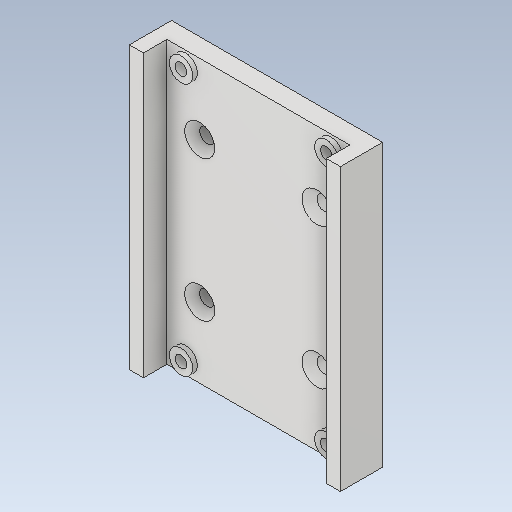
# Autodesk Inventor part: 회로프레임
Saved by Autodesk Inventor 2020.5 (Build 245400000, 400)
## iProperties
Created: 2021-07-21
Part Number: 회로프레임
Material: LCP 플라스틱
Document SubType Name: Modeling
Designer: user
Density: 1.626 g/cm^3
Appearance: 매끄러움 - 흰색
Mass: 20.1348 g
Surface Area: 77.5279 cm^2
Volume: 12.3831 cm^3
Author: user
Autodesk Inventor part; units mm, degrees
ref_plane "YZ Plane" through (0, 0, 0) normal (1, 0, 0) x (0, 1, 0)
ref_plane "XZ Plane" through (0, 0, 0) normal (0, 1, 0) x (-1, 0, 0)
ref_plane "XY Plane" through (0, 0, 0) normal (0, 0, 1) x (1, 0, 0)
sketch "스케치1" plane through (0, 0, 0) normal (0, 0, 1) x (1, 0, 0)
  line L0 (-22.5, 30) -> (22.5, 30)
  line L1 (22.5, 30) -> (22.5, -30)
  line L2 (22.5, -30) -> (-22.5, -30)
  line L3 (-22.5, -30) -> (-22.5, 30)
  point P0 (0, 0)
  dimension "d0" = 45
  dimension "d1" = 60
  dimension "d2" = 30
  dimension "d3" = 22.5
  constraints: 8 end point, 2 parallel, 1 horizontal, 1 perpendicular
  measures "d0" distance of L1.end L2.end
  measures "d1" distance of L0.end L1.end
  measures "d2" distance from line of L0 point (0, 0)
  measures "d3" distance from line of L3 point (0, 0)
extrude "돌출1" add sketch "스케치1" along normal blind 4
sketch "스케치2" plane through (0, 0, 4) normal (0, 0, 1) x (1, 0, 0)
  line L0 (-15.5, 27) -> (15.5, 27)
  line L1 (15.5, 27) -> (15.5, -27)
  line L2 (15.5, -27) -> (-15.5, -27)
  line L3 (-15.5, -27) -> (-15.5, 27)
  circle A0 centre (-15.5, 27) radius 1.25
  circle A1 centre (15.5, 27) radius 1.25
  circle A2 centre (-15.5, -27) radius 1.25
  circle A3 centre (15.5, -27) radius 1.25
  point P0 (0, 0)
  dimension "d6" = 31
  dimension "d7" = 54
  dimension "d8" = 15.5
  dimension "d9" = 27
  dimension "d10" = 2.5
  dimension "d11" = 2.5
  dimension "d12" = 2.5
  dimension "d13" = 2.5
  constraints: 8 end point, 4 centre point, 4 coincident, 2 parallel, 1 horizontal, 1 perpendicular
  measures "d6" distance between parallel lines of L1 L3
  measures "d7" distance between parallel lines of L2 L0
  measures "d8" distance from line of L3 point (0, 0)
  measures "d9" distance from line of point (0, 0) L0
  measures "d10" diameter of A0
  measures "d11" diameter of A1
  measures "d12" diameter of A2
  measures "d13" diameter of A3
extrude "돌출2" cut sketch "스케치2" against normal up to surface (4 mm away) contours L3 A0 L0 | L0 A0 L3 | A1 L1 L0 | L0 L1 A1 | A2 L2 L3 | L3 L2 A2 | A3 L2 L1 | L1 L2 A3
sketch "스케치3" plane through (0, 0, 4) normal (0, 0, 1) x (1, 0, 0)
  line L0 (-22.5, 30) -> (-22.5, -30) projected
  line L1 (-22.5, -30) -> (22.5, -30) projected
  line L2 (-22.5, 30) -> (-19.5, 30)
  line L3 (-19.5, 30) -> (-19.5, -30)
  line L4 (-19.5, -30) -> (-22.5, -30)
  line L5 (-22.5, -30) -> (-22.5, 30)
  line L6 (22.5, 30) -> (-22.5, 30) projected
  line L7 (22.5, 30) -> (19.5, 30)
  line L8 (19.5, 30) -> (19.5, -30)
  line L9 (19.5, -30) -> (22.5, -30)
  line L10 (22.5, -30) -> (22.5, 30)
  point P0 (0, 0)
  dimension "d16" = 3
  dimension "d17" = 3
  constraints: 16 end point, 4 parallel, 2 horizontal, 2 perpendicular, 2 point on line
  measures "d16" distance between parallel lines of L3 L0
  measures "d17" distance between parallel lines of L10 L8
extrude "돌출3" add sketch "스케치3" along normal blind 5 contours L2 L3 L1 L0 | L6 L10 L1 L8
sketch "스케치4" plane through (0, 0, 4) normal (0, 0, 1) x (1, 0, 0)
  circle A0 centre (-15.5, 27) radius 1.25 projected
  circle A1 centre (15.5, 27) radius 1.25 projected
  circle A2 centre (15.5, -27) radius 1.25 projected
  circle A3 centre (-15.5, -27) radius 1.25 projected
  circle A4 centre (-15.5, 27) radius 2.5
  circle A5 centre (-15.5, 27) radius 1.25
  circle A6 centre (15.5, 27) radius 2.5
  circle A7 centre (15.5, 27) radius 1.25
  circle A8 centre (15.5, -27) radius 2.5
  circle A9 centre (15.5, -27) radius 1.25
  circle A10 centre (-15.5, -27) radius 2.5
  circle A11 centre (-15.5, -27) radius 1.25
  point P0 (0, 0)
  dimension "d20" = 5
  dimension "d21" = 2.5
  dimension "d22" = 5
  dimension "d23" = 2.5
  dimension "d24" = 5
  dimension "d25" = 2.5
  dimension "d26" = 5
  dimension "d27" = 2.5
  constraints: 8 centre point, 8 coincident
  measures "d20" diameter of A4
  measures "d21" diameter of A5
  measures "d22" diameter of A6
  measures "d23" diameter of A7
  measures "d24" diameter of A8
  measures "d25" diameter of A9
  measures "d26" diameter of A10
  measures "d27" diameter of A11
extrude "돌출4" add sketch "스케치4" along normal blind 1
sketch "스케치5" plane through (0, 0, 4) normal (0, 0, 1) x (1, 0, 0)
  line L0 (-12.5, 15) -> (12.5, 15)
  line L1 (12.5, 15) -> (12.5, -15)
  line L2 (12.5, -15) -> (-12.5, -15)
  line L3 (-12.5, -15) -> (-12.5, 15)
  circle A0 centre (-12.5, 15) radius 1.6
  circle A1 centre (12.5, 15) radius 1.6
  circle A2 centre (-12.5, -15) radius 1.6
  circle A3 centre (12.5, -15) radius 1.6
  point P0 (0, 0)
  dimension "d30" = 25
  dimension "d31" = 30
  dimension "d32" = 15
  dimension "d33" = 12.5
  dimension "d34" = 3.2
  dimension "d35" = 3.2
  dimension "d36" = 3.2
  dimension "d37" = 3.2
  constraints: 8 end point, 4 centre point, 4 coincident, 2 parallel, 1 horizontal, 1 perpendicular
  measures "d30" distance of L1.end L2.end
  measures "d31" distance of L0.end L1.end
  measures "d32" distance from line of L0 point (0, 0)
  measures "d33" distance from line of point (0, 0) L1
  measures "d34" diameter of A0
  measures "d35" diameter of A1
  measures "d36" diameter of A2
  measures "d37" diameter of A3
extrude "돌출5" cut sketch "스케치5" against normal up to surface (4 mm away) contours L3 A0 L0 | L0 A0 L3 | A1 L1 L0 | L0 L1 A1 | A2 L2 L3 | L3 L2 A2 | A3 L2 L1 | L1 L2 A3
chamfer "모따기1" distance 1.6 angle 45 4 edges at (10.9, -15, 4) (-14.1, -15, 4) (10.9, 15, 4) (-14.1, 15, 4)
equation "\"d2\" = 0.5 * d1"
equation "\"d3\" = 0.5 * d0"
equation "\"d8\" = 0.5 * d6"
equation "\"d9\" = 0.5 * d7"
equation "\"d32\" = 0.5 * d31"
equation "\"d33\" = 0.5 * d30"
